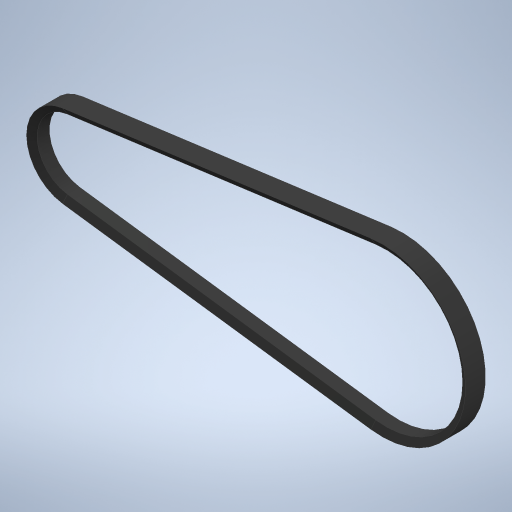
# Autodesk Inventor part: Dây đai
Saved by Autodesk Inventor 2023 (Build 270158000, 158)
## iProperties
Created: 2023-10-09
Part Number: Dây đai
Material: Generic
Document SubType Name: Modeling
Designer: huy20
Density: 1 g/cm^3
Appearance: Default
Author: huy20
Autodesk Inventor part; units mm, degrees
ref_plane "YZ Plane" through (0, 0, 0) normal (1, 0, 0) x (0, 1, 0)
ref_plane "XZ Plane" through (0, 0, 0) normal (0, 1, 0) x (-1, 0, 0)
sketch "Sketch1" plane through (0, 0, 0) normal (0, 0, 1) x (1, 0, 0)
  arc A0 (-3.0584, -22.7957) -> (-3.0593, 22.7956) centre (0, 0) ccw
  arc A1 (-95.3861, 10.4049) -> (-95.3857, -10.4086) centre (-93.9895, -0.0018) ccw
  line L0 (-95.3861, 10.4049) -> (-3.0593, 22.7956)
  line L1 (-95.3857, -10.4086) -> (-3.0584, -22.7957)
  dimension "d0" = 46
  dimension "d1" = 21
  constraints: 4 end point, 4 point on circle, 4 tangent, 2 centre point, 1 coincident
  measures "d0" diameter of A0
  measures "d1" diameter of A1
ref_plane "Work Plane1" through (-3.0593, 22.7956, 0) normal (-0.9911143, -0.1330127, 0) x (0.1330127, -0.9911143, 0)
sketch "Sketch2" plane through (-3.0593, 22.7956, 0) normal (-0.9911143, -0.1330127, 0) x (0.1330127, -0.9911143, 0)
  line L0 (-2, 0) -> (-2, 3)
  line L1 (-2, 0) -> (-2, -3)
  line L2 (-2, -3) -> (0, -1.8453)
  line L3 (0, -1.8453) -> (0, 1.8453)
  line L4 (0, 1.8453) -> (-2, 3)
  point P0 (23, 0)
  dimension "d4" = 3
  dimension "d5" = 3
  dimension "d6" = 60
  dimension "d7" = 60
  dimension "d8" = 2
  constraints: 10 end point, 1 parallel, 1 vertical
  measures "d4" distance of L0.start L0.end
  measures "d5" distance of L0.start L1.end
  measures "d6" angle of L4 L0
  measures "d7" angle of L1 L2
  measures "d8" distance between parallel lines of L3 L0
sweep "Sweep1" add profiles "Sketch2" path "Sketch1"
body "Solid1"
